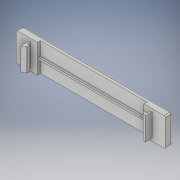
# Autodesk Inventor part: ClipMale
Saved by Autodesk Inventor 2019 (Build 230136000, 136)
## iProperties
Created: 2019-01-05
Part Number: ClipMale
Material: Generic
Document SubType Name: Modeling
Designer: Nate
Density: 1 g/cm^3
Appearance: Default
Author: Nate
Autodesk Inventor part; units mm, degrees
ref_plane "YZ Plane" through (0, 0, 0) normal (1, 0, 0) x (0, 1, 0)
ref_plane "XZ Plane" through (0, 0, 0) normal (0, 1, 0) x (-1, 0, 0)
ref_plane "XY Plane" through (0, 0, 0) normal (0, 0, 1) x (1, 0, 0)
sketch "Sketch1" plane through (0, 0, 0) normal (0, 0, 1) x (1, 0, 0)
  line L0 (0, 0) -> (66.675, 0)
  line L1 (66.675, 0) -> (66.675, -12.7)
  line L2 (66.675, -12.7) -> (0, -12.7)
  line L3 (0, -12.7) -> (0, 0)
  dimension "d0" = 66.675
  dimension "d1" = 12.7
  constraints: 8 end point, 2 parallel, 1 horizontal, 1 perpendicular
  measures "d0" distance of L1.end L2.end
  measures "d1" distance of L0.end L1.end
extrude "Extrusion1" add sketch "Sketch1" along normal blind 3.175
fillet "Fillet1" radius 0.635 8 edges at (33.3375, 0, 0) (66.675, -6.35, 0) (66.675, 0, 1.5875) (33.3375, -12.7, 0) (66.675, -12.7, 1.5875) (0, -6.35, 0) (0, -12.7, 1.5875) (0, 0, 1.5875)
sketch "Sketch2" plane through (0, 0, 3.175) normal (0, 0, 1) x (1, 0, 0)
  line L0 (66.04, 0) -> (0.635, 0) projected
  line L1 (0.635, -12.7) -> (66.04, -12.7) projected
  line L2 (9.525, 0) -> (57.15, 0)
  line L3 (57.15, 0) -> (57.15, -12.7)
  line L4 (57.15, -12.7) -> (9.525, -12.7)
  line L5 (9.525, -12.7) -> (9.525, 0)
  line L6 (66.675, -12.065) -> (66.675, -0.635) projected
  point P0 (0, 0)
  dimension "d5" = 47.625
  dimension "d6" = 9.525
  constraints: 8 end point, 2 parallel, 2 point on line, 1 horizontal, 1 perpendicular
  measures "d5" distance of L3.end L4.end
  measures "d6" distance between parallel lines of L6 L3
extrude "Extrusion2" cut sketch "Sketch2" against normal blind 1.397
sketch "Sketch3" plane through (0, 0, 3.175) normal (0, 0, 1) x (1, 0, 0)
  line L0 (66.04, -0.635) -> (0.635, -0.635) projected
  line L1 (0.635, -12.065) -> (66.04, -12.065) projected
  line L2 (5.842, -1.27) -> (7.62, -1.27)
  line L3 (7.62, -1.27) -> (7.62, -11.43)
  line L4 (7.62, -11.43) -> (5.842, -11.43)
  line L5 (5.842, -11.43) -> (5.842, -1.27)
  line L6 (9.525, -12.7) -> (9.525, 0) projected
  line L7 (7.112, -1.101) -> (5.842, -11.4757)
  line L8 (5.842, -11.4757) -> (8.89, -11.4757)
  line L9 (8.89, -11.4757) -> (7.62, -21.8503)
  line L10 (9.525, 0) -> (0.635, 0) projected
  line L11 (0.635, -12.7) -> (9.525, -12.7) projected
  point P0 (0, 0)
  dimension "d9" = 1.778
  dimension "d52" = 1.27
  dimension "d53" = 1.27
  dimension "d56" = 1.905
  constraints: 14 end point, 3 parallel, 2 point on line, 1 horizontal, 1 perpendicular
  measures "d9" distance between parallel lines of L5 L3
  measures "d52" distance from line of L10 L2.end
  measures "d53" distance from line of L11 L4.end
  measures "d56" distance from line of L6.end L3
extrude "Extrusion3" add sketch "Sketch3" along normal blind 3.81 contours L4 L5 L2 L7 | L7 L2 L3 L4
sketch "Sketch5" plane through (0, 0, 3.175) normal (0, 0, 1) x (1, 0, 0)
  line L0 (66.04, -0.635) -> (0.635, -0.635) projected
  line L1 (0.635, -12.065) -> (66.04, -12.065) projected
  line L2 (59.055, -1.27) -> (60.833, -1.27)
  line L3 (60.833, -1.27) -> (60.833, -11.43)
  line L4 (60.833, -11.43) -> (59.055, -11.43)
  line L5 (59.055, -11.43) -> (59.055, -1.27)
  line L6 (57.15, 0) -> (57.15, -12.7) projected
  line L7 (66.04, 0) -> (57.15, 0) projected
  line L8 (57.15, -12.7) -> (66.04, -12.7) projected
  point P0 (0, 0)
  dimension "d21" = 1.778
  dimension "d54" = 1.27
  dimension "d55" = 1.27
  dimension "d57" = 1.905
  constraints: 8 end point, 2 parallel, 1 horizontal, 1 perpendicular
  measures "d21" distance of L3.end L4.end
  measures "d54" distance from line of L7 L2.end
  measures "d55" distance from line of L8 L4.end
  measures "d57" distance between parallel lines of L6 L5
extrude "Extrusion5" add sketch "Sketch5" along normal blind 3.175
sketch "Sketch6" plane through (59.055, -1.27, 3.175) normal (0, 1, 0) x (1, 0, 0)
  line L0 (0, 0) -> (1.778, 0) projected
  line L1 (1.016, -1.524) -> (1.016, 0)
  line L2 (1.016, 0) -> (0, 0)
  line L3 (0, 0) -> (0, -1.524)
  line L4 (0, 0) -> (0, -3.175) projected
  line L5 (0, 0) -> (1.016, 0)
  line L6 (1.016, 0) -> (1.016, -1.524)
  line L7 (1.016, -1.524) -> (0, -1.524)
  line L8 (0, -1.524) -> (0, 0)
  point P0 (-59.055, 3.175)
  point P1 (0, -1.524)
  dimension "d29" = 1.016
  dimension "d51" = 1.524
  constraints: 14 end point, 3 parallel, 1 collinear, 1 horizontal, 1 perpendicular, 1 point on line
  measures "d29" distance between parallel lines of L3 L1
  measures "d51" distance of L2.end L3.end
extrude "Extrusion6" cut sketch "Sketch6" against normal through all
sketch "Sketch7" plane through (0, 0, 1.778) normal (0, 0, 1) x (1, 0, 0)
  line L0 (9.525, -12.7) -> (9.525, 0) projected
  line L1 (57.15, 0) -> (57.15, -12.7) projected
  line L2 (9.525, -5.9055) -> (57.15, -5.9055)
  line L3 (57.15, -5.9055) -> (57.15, -6.7945)
  line L4 (57.15, -6.7945) -> (9.525, -6.7945)
  line L5 (9.525, -6.7945) -> (9.525, -5.9055)
  line L6 (9.525, 0) -> (57.15, 0) projected
  point P0 (0, 0)
  dimension "d33" = 0.889
  dimension "d34" = 5.9055
  constraints: 8 end point, 2 parallel, 2 point on line, 1 horizontal, 1 perpendicular
  measures "d33" distance of L2.end L3.end
  measures "d34" distance between parallel lines of L6 L2
extrude "Extrusion7" add sketch "Sketch7" along normal blind 1.016 contours L0 L2 L1 L4
sketch "Sketch8" plane through (5.842, -1.27, 3.175) normal (0, 1, 0) x (1, 0, 0)
  line L0 (0, 0) -> (1.778, 0) projected
  line L1 (1.778, 0) -> (0.762, 0)
  line L2 (0.762, 0) -> (0.762, -1.524)
  line L3 (0.762, -1.524) -> (1.778, -1.524)
  line L4 (1.778, -1.524) -> (1.778, 0)
  point P0 (-5.842, 3.175)
  dimension "d38" = 1.016
  dimension "d39" = 1.524
  constraints: 8 end point, 2 parallel, 1 collinear, 1 horizontal, 1 perpendicular
  measures "d38" distance of L3.end L2.end
  measures "d39" distance of L2.end L1.end
extrude "Extrusion8" cut sketch "Sketch8" against normal through all
chamfer "Chamfer3" distance 1.778 angle 30 1 edges at (7.62, -6.35, 6.985) measured on face at (6.4347, -4.6567, 6.985)
fillet "Fillet4" radius 0.3175 1 edges at (7.62, -6.35, 5.959)
chamfer "Chamfer4" distance 1.778 angle 25 1 edges at (59.055, -6.35, 6.35) measured on face at (59.6477, -4.6567, 6.35)
fillet "Fillet5" radius 0.3175 1 edges at (59.055, -6.35, 5.5214)
body "Solid1"
